Autodesk Fusion 360 part; units mm, degrees
(part 2 of 4)
  spline S79 degree 3 poles (-131.9897, -42.366) (-131.3663, -43.0785) (-131.0085, -44.0182) (-131.0002, -44.9649) (-130.9916, -45.935) (-131.3508, -46.9039) (-131.9897, -47.634) knots -1 -1 -1 -1 -0.506107 -0.506107 -0.506107 0 0 0 0
  spline S80 degree 3 poles (-131.9897, -37.634) (-132.7286, -38.4785) (-133.8364, -38.9881) (-134.9584, -38.9998) (-136.1081, -39.0117) (-137.2531, -38.4994) (-138.0103, -37.634) knots -1 -1 -1 -1 -0.506107 -0.506107 -0.506107 0 0 0 0
  spline S81 degree 3 poles (-138.0103, -37.634) (-138.6337, -36.9215) (-138.9915, -35.9818) (-138.9998, -35.0351) (-139.0084, -34.065) (-138.6492, -33.0961) (-138.0103, -32.366) knots -1 -1 -1 -1 -0.506107 -0.506107 -0.506107 0 0 0 0
  spline S82 degree 3 poles (-138.0103, -32.366) (-137.2714, -31.5215) (-136.1636, -31.0119) (-135.0416, -31.0002) (-133.8919, -30.9883) (-132.7469, -31.5006) (-131.9897, -32.366) knots -1 -1 -1 -1 -0.506107 -0.506107 -0.506107 0 0 0 0
  spline S83 degree 3 poles (-131.9897, -32.366) (-131.3663, -33.0785) (-131.0085, -34.0182) (-131.0002, -34.9649) (-130.9916, -35.935) (-131.3508, -36.9039) (-131.9897, -37.634) knots -1 -1 -1 -1 -0.506107 -0.506107 -0.506107 0 0 0 0
  spline S84 degree 3 poles (-131.9897, -27.634) (-132.7286, -28.4785) (-133.8364, -28.9881) (-134.9584, -28.9998) (-136.1081, -29.0117) (-137.2531, -28.4994) (-138.0103, -27.634) knots -1 -1 -1 -1 -0.506107 -0.506107 -0.506107 0 0 0 0
  spline S85 degree 3 poles (-138.0103, -27.634) (-138.6337, -26.9215) (-138.9915, -25.9818) (-138.9998, -25.0351) (-139.0084, -24.065) (-138.6492, -23.0961) (-138.0103, -22.366) knots -1 -1 -1 -1 -0.506107 -0.506107 -0.506107 0 0 0 0
  spline S86 degree 3 poles (-138.0103, -22.366) (-137.2714, -21.5215) (-136.1636, -21.0119) (-135.0416, -21.0002) (-133.8919, -20.9883) (-132.7469, -21.5006) (-131.9897, -22.366) knots -1 -1 -1 -1 -0.506107 -0.506107 -0.506107 0 0 0 0
  spline S87 degree 3 poles (-131.9897, -22.366) (-131.3663, -23.0785) (-131.0085, -24.0182) (-131.0002, -24.9649) (-130.9916, -25.935) (-131.3508, -26.9039) (-131.9897, -27.634) knots -1 -1 -1 -1 -0.506107 -0.506107 -0.506107 0 0 0 0
  spline S88 degree 3 poles (-131.9897, -17.634) (-132.7286, -18.4785) (-133.8364, -18.9881) (-134.9584, -18.9998) (-136.1081, -19.0117) (-137.2531, -18.4994) (-138.0103, -17.634) knots -1 -1 -1 -1 -0.506107 -0.506107 -0.506107 0 0 0 0
  spline S89 degree 3 poles (-138.0103, -17.634) (-138.6337, -16.9215) (-138.9915, -15.9818) (-138.9998, -15.0351) (-139.0084, -14.065) (-138.6492, -13.0961) (-138.0103, -12.366) knots -1 -1 -1 -1 -0.506107 -0.506107 -0.506107 0 0 0 0
  spline S90 degree 3 poles (-138.0103, -12.366) (-137.2714, -11.5215) (-136.1636, -11.0119) (-135.0416, -11.0002) (-133.8919, -10.9883) (-132.7469, -11.5006) (-131.9897, -12.366) knots -1 -1 -1 -1 -0.506107 -0.506107 -0.506107 0 0 0 0
  spline S91 degree 3 poles (-131.9897, -12.366) (-131.3663, -13.0785) (-131.0085, -14.0182) (-131.0002, -14.9649) (-130.9916, -15.935) (-131.3508, -16.9039) (-131.9897, -17.634) knots -1 -1 -1 -1 -0.506107 -0.506107 -0.506107 0 0 0 0
  spline S92 degree 3 poles (-131.9897, -7.634) (-132.7286, -8.4785) (-133.8364, -8.9881) (-134.9584, -8.9998) (-136.1081, -9.0117) (-137.2531, -8.4994) (-138.0103, -7.634) knots -1 -1 -1 -1 -0.506107 -0.506107 -0.506107 0 0 0 0
  spline S93 degree 3 poles (-138.0103, -7.634) (-138.6337, -6.9215) (-138.9915, -5.9818) (-138.9998, -5.0351) (-139.0084, -4.065) (-138.6492, -3.0961) (-138.0103, -2.366) knots -1 -1 -1 -1 -0.506107 -0.506107 -0.506107 0 0 0 0
  spline S94 degree 3 poles (-138.0103, -2.366) (-137.2714, -1.5215) (-136.1636, -1.0119) (-135.0416, -1.0002) (-133.8919, -0.9883) (-132.7469, -1.5006) (-131.9897, -2.366) knots -1 -1 -1 -1 -0.506107 -0.506107 -0.506107 0 0 0 0
  spline S95 degree 3 poles (-131.9897, -2.366) (-131.3663, -3.0785) (-131.0085, -4.0182) (-131.0002, -4.9649) (-130.9916, -5.935) (-131.3508, -6.9039) (-131.9897, -7.634) knots -1 -1 -1 -1 -0.506107 -0.506107 -0.506107 0 0 0 0
  spline S96 degree 3 poles (-121.9897, -77.634) (-122.7286, -78.4785) (-123.8364, -78.9881) (-124.9584, -78.9998) (-126.1081, -79.0117) (-127.2531, -78.4994) (-128.0103, -77.634) knots -1 -1 -1 -1 -0.506107 -0.506107 -0.506107 0 0 0 0
  spline S97 degree 3 poles (-128.0103, -77.634) (-128.6337, -76.9215) (-128.9915, -75.9818) (-128.9998, -75.0351) (-129.0084, -74.065) (-128.6492, -73.0961) (-128.0103, -72.366) knots -1 -1 -1 -1 -0.506107 -0.506107 -0.506107 0 0 0 0
  spline S98 degree 3 poles (-128.0103, -72.366) (-127.2714, -71.5215) (-126.1636, -71.0119) (-125.0416, -71.0002) (-123.8919, -70.9883) (-122.7469, -71.5006) (-121.9897, -72.366) knots -1 -1 -1 -1 -0.506107 -0.506107 -0.506107 0 0 0 0
  spline S99 degree 3 poles (-121.9897, -72.366) (-121.3663, -73.0785) (-121.0085, -74.0182) (-121.0002, -74.9649) (-120.9916, -75.935) (-121.3508, -76.9039) (-121.9897, -77.634) knots -1 -1 -1 -1 -0.506107 -0.506107 -0.506107 0 0 0 0
  spline S100 degree 3 poles (-121.9897, -67.634) (-122.7286, -68.4785) (-123.8364, -68.9881) (-124.9584, -68.9998) (-126.1081, -69.0117) (-127.2531, -68.4994) (-128.0103, -67.634) knots -1 -1 -1 -1 -0.506107 -0.506107 -0.506107 0 0 0 0
  spline S101 degree 3 poles (-128.0103, -67.634) (-128.6337, -66.9215) (-128.9915, -65.9818) (-128.9998, -65.0351) (-129.0084, -64.065) (-128.6492, -63.0961) (-128.0103, -62.366) knots -1 -1 -1 -1 -0.506107 -0.506107 -0.506107 0 0 0 0
  spline S102 degree 3 poles (-128.0103, -62.366) (-127.2714, -61.5215) (-126.1636, -61.0119) (-125.0416, -61.0002) (-123.8919, -60.9883) (-122.7469, -61.5006) (-121.9897, -62.366) knots -1 -1 -1 -1 -0.506107 -0.506107 -0.506107 0 0 0 0
  spline S103 degree 3 poles (-121.9897, -62.366) (-121.3663, -63.0785) (-121.0085, -64.0182) (-121.0002, -64.9649) (-120.9916, -65.935) (-121.3508, -66.9039) (-121.9897, -67.634) knots -1 -1 -1 -1 -0.506107 -0.506107 -0.506107 0 0 0 0
  spline S104 degree 3 poles (-121.9897, -57.634) (-122.7286, -58.4785) (-123.8364, -58.9881) (-124.9584, -58.9998) (-126.1081, -59.0117) (-127.2531, -58.4994) (-128.0103, -57.634) knots -1 -1 -1 -1 -0.506107 -0.506107 -0.506107 0 0 0 0
  spline S105 degree 3 poles (-128.0103, -57.634) (-128.6337, -56.9215) (-128.9915, -55.9818) (-128.9998, -55.0351) (-129.0084, -54.065) (-128.6492, -53.0961) (-128.0103, -52.366) knots -1 -1 -1 -1 -0.506107 -0.506107 -0.506107 0 0 0 0
  spline S106 degree 3 poles (-128.0103, -52.366) (-127.2714, -51.5215) (-126.1636, -51.0119) (-125.0416, -51.0002) (-123.8919, -50.9883) (-122.7469, -51.5006) (-121.9897, -52.366) knots -1 -1 -1 -1 -0.506107 -0.506107 -0.506107 0 0 0 0
  spline S107 degree 3 poles (-121.9897, -52.366) (-121.3663, -53.0785) (-121.0085, -54.0182) (-121.0002, -54.9649) (-120.9916, -55.935) (-121.3508, -56.9039) (-121.9897, -57.634) knots -1 -1 -1 -1 -0.506107 -0.506107 -0.506107 0 0 0 0
  spline S108 degree 3 poles (-121.9897, -47.634) (-122.7286, -48.4785) (-123.8364, -48.9881) (-124.9584, -48.9998) (-126.1081, -49.0117) (-127.2531, -48.4994) (-128.0103, -47.634) knots -1 -1 -1 -1 -0.506107 -0.506107 -0.506107 0 0 0 0
  spline S109 degree 3 poles (-128.0103, -47.634) (-128.6337, -46.9215) (-128.9915, -45.9818) (-128.9998, -45.0351) (-129.0084, -44.065) (-128.6492, -43.0961) (-128.0103, -42.366) knots -1 -1 -1 -1 -0.506107 -0.506107 -0.506107 0 0 0 0
  spline S110 degree 3 poles (-128.0103, -42.366) (-127.2714, -41.5215) (-126.1636, -41.0119) (-125.0416, -41.0002) (-123.8919, -40.9883) (-122.7469, -41.5006) (-121.9897, -42.366) knots -1 -1 -1 -1 -0.506107 -0.506107 -0.506107 0 0 0 0
  spline S111 degree 3 poles (-121.9897, -42.366) (-121.3663, -43.0785) (-121.0085, -44.0182) (-121.0002, -44.9649) (-120.9916, -45.935) (-121.3508, -46.9039) (-121.9897, -47.634) knots -1 -1 -1 -1 -0.506107 -0.506107 -0.506107 0 0 0 0
  spline S112 degree 3 poles (-121.9897, -37.634) (-122.7286, -38.4785) (-123.8364, -38.9881) (-124.9584, -38.9998) (-126.1081, -39.0117) (-127.2531, -38.4994) (-128.0103, -37.634) knots -1 -1 -1 -1 -0.506107 -0.506107 -0.506107 0 0 0 0
  spline S113 degree 3 poles (-128.0103, -37.634) (-128.6337, -36.9215) (-128.9915, -35.9818) (-128.9998, -35.0351) (-129.0084, -34.065) (-128.6492, -33.0961) (-128.0103, -32.366) knots -1 -1 -1 -1 -0.506107 -0.506107 -0.506107 0 0 0 0
  spline S114 degree 3 poles (-128.0103, -32.366) (-127.2714, -31.5215) (-126.1636, -31.0119) (-125.0416, -31.0002) (-123.8919, -30.9883) (-122.7469, -31.5006) (-121.9897, -32.366) knots -1 -1 -1 -1 -0.506107 -0.506107 -0.506107 0 0 0 0
  spline S115 degree 3 poles (-121.9897, -32.366) (-121.3663, -33.0785) (-121.0085, -34.0182) (-121.0002, -34.9649) (-120.9916, -35.935) (-121.3508, -36.9039) (-121.9897, -37.634) knots -1 -1 -1 -1 -0.506107 -0.506107 -0.506107 0 0 0 0
  spline S116 degree 3 poles (-121.9897, -27.634) (-122.7286, -28.4785) (-123.8364, -28.9881) (-124.9584, -28.9998) (-126.1081, -29.0117) (-127.2531, -28.4994) (-128.0103, -27.634) knots -1 -1 -1 -1 -0.506107 -0.506107 -0.506107 0 0 0 0
  spline S117 degree 3 poles (-128.0103, -27.634) (-128.6337, -26.9215) (-128.9915, -25.9818) (-128.9998, -25.0351) (-129.0084, -24.065) (-128.6492, -23.0961) (-128.0103, -22.366) knots -1 -1 -1 -1 -0.506107 -0.506107 -0.506107 0 0 0 0
  spline S118 degree 3 poles (-128.0103, -22.366) (-127.2714, -21.5215) (-126.1636, -21.0119) (-125.0416, -21.0002) (-123.8919, -20.9883) (-122.7469, -21.5006) (-121.9897, -22.366) knots -1 -1 -1 -1 -0.506107 -0.506107 -0.506107 0 0 0 0
  spline S119 degree 3 poles (-121.9897, -22.366) (-121.3663, -23.0785) (-121.0085, -24.0182) (-121.0002, -24.9649) (-120.9916, -25.935) (-121.3508, -26.9039) (-121.9897, -27.634) knots -1 -1 -1 -1 -0.506107 -0.506107 -0.506107 0 0 0 0
  spline S120 degree 3 poles (-121.9897, -17.634) (-122.7286, -18.4785) (-123.8364, -18.9881) (-124.9584, -18.9998) (-126.1081, -19.0117) (-127.2531, -18.4994) (-128.0103, -17.634) knots -1 -1 -1 -1 -0.506107 -0.506107 -0.506107 0 0 0 0
  spline S121 degree 3 poles (-128.0103, -17.634) (-128.6337, -16.9215) (-128.9915, -15.9818) (-128.9998, -15.0351) (-129.0084, -14.065) (-128.6492, -13.0961) (-128.0103, -12.366) knots -1 -1 -1 -1 -0.506107 -0.506107 -0.506107 0 0 0 0
  spline S122 degree 3 poles (-128.0103, -12.366) (-127.2714, -11.5215) (-126.1636, -11.0119) (-125.0416, -11.0002) (-123.8919, -10.9883) (-122.7469, -11.5006) (-121.9897, -12.366) knots -1 -1 -1 -1 -0.506107 -0.506107 -0.506107 0 0 0 0
  spline S123 degree 3 poles (-121.9897, -12.366) (-121.3663, -13.0785) (-121.0085, -14.0182) (-121.0002, -14.9649) (-120.9916, -15.935) (-121.3508, -16.9039) (-121.9897, -17.634) knots -1 -1 -1 -1 -0.506107 -0.506107 -0.506107 0 0 0 0
  spline S124 degree 3 poles (-121.9897, -7.634) (-122.7286, -8.4785) (-123.8364, -8.9881) (-124.9584, -8.9998) (-126.1081, -9.0117) (-127.2531, -8.4994) (-128.0103, -7.634) knots -1 -1 -1 -1 -0.506107 -0.506107 -0.506107 0 0 0 0
  spline S125 degree 3 poles (-128.0103, -7.634) (-128.6337, -6.9215) (-128.9915, -5.9818) (-128.9998, -5.0351) (-129.0084, -4.065) (-128.6492, -3.0961) (-128.0103, -2.366) knots -1 -1 -1 -1 -0.506107 -0.506107 -0.506107 0 0 0 0
  spline S126 degree 3 poles (-128.0103, -2.366) (-127.2714, -1.5215) (-126.1636, -1.0119) (-125.0416, -1.0002) (-123.8919, -0.9883) (-122.7469, -1.5006) (-121.9897, -2.366) knots -1 -1 -1 -1 -0.506107 -0.506107 -0.506107 0 0 0 0
  spline S127 degree 3 poles (-121.9897, -2.366) (-121.3663, -3.0785) (-121.0085, -4.0182) (-121.0002, -4.9649) (-120.9916, -5.935) (-121.3508, -6.9039) (-121.9897, -7.634) knots -1 -1 -1 -1 -0.506107 -0.506107 -0.506107 0 0 0 0
  spline S128 degree 3 poles (-111.9897, -77.634) (-112.7286, -78.4785) (-113.8364, -78.9881) (-114.9584, -78.9998) (-116.1081, -79.0117) (-117.2531, -78.4994) (-118.0103, -77.634) knots -1 -1 -1 -1 -0.506107 -0.506107 -0.506107 0 0 0 0
  spline S129 degree 3 poles (-118.0103, -77.634) (-118.6337, -76.9215) (-118.9915, -75.9818) (-118.9998, -75.0351) (-119.0084, -74.065) (-118.6492, -73.0961) (-118.0103, -72.366) knots -1 -1 -1 -1 -0.506107 -0.506107 -0.506107 0 0 0 0
  spline S130 degree 3 poles (-118.0103, -72.366) (-117.2714, -71.5215) (-116.1636, -71.0119) (-115.0416, -71.0002) (-113.8919, -70.9883) (-112.7469, -71.5006) (-111.9897, -72.366) knots -1 -1 -1 -1 -0.506107 -0.506107 -0.506107 0 0 0 0
  spline S131 degree 3 poles (-111.9897, -72.366) (-111.3663, -73.0785) (-111.0085, -74.0182) (-111.0002, -74.9649) (-110.9916, -75.935) (-111.3508, -76.9039) (-111.9897, -77.634) knots -1 -1 -1 -1 -0.506107 -0.506107 -0.506107 0 0 0 0
  spline S132 degree 3 poles (-111.9897, -67.634) (-112.7286, -68.4785) (-113.8364, -68.9881) (-114.9584, -68.9998) (-116.1081, -69.0117) (-117.2531, -68.4994) (-118.0103, -67.634) knots -1 -1 -1 -1 -0.506107 -0.506107 -0.506107 0 0 0 0
  spline S133 degree 3 poles (-118.0103, -67.634) (-118.6337, -66.9215) (-118.9915, -65.9818) (-118.9998, -65.0351) (-119.0084, -64.065) (-118.6492, -63.0961) (-118.0103, -62.366) knots -1 -1 -1 -1 -0.506107 -0.506107 -0.506107 0 0 0 0
  spline S134 degree 3 poles (-118.0103, -62.366) (-117.2714, -61.5215) (-116.1636, -61.0119) (-115.0416, -61.0002) (-113.8919, -60.9883) (-112.7469, -61.5006) (-111.9897, -62.366) knots -1 -1 -1 -1 -0.506107 -0.506107 -0.506107 0 0 0 0
  spline S135 degree 3 poles (-111.9897, -62.366) (-111.3663, -63.0785) (-111.0085, -64.0182) (-111.0002, -64.9649) (-110.9916, -65.935) (-111.3508, -66.9039) (-111.9897, -67.634) knots -1 -1 -1 -1 -0.506107 -0.506107 -0.506107 0 0 0 0
  spline S136 degree 3 poles (-111.9897, -57.634) (-112.7286, -58.4785) (-113.8364, -58.9881) (-114.9584, -58.9998) (-116.1081, -59.0117) (-117.2531, -58.4994) (-118.0103, -57.634) knots -1 -1 -1 -1 -0.506107 -0.506107 -0.506107 0 0 0 0
  spline S137 degree 3 poles (-118.0103, -57.634) (-118.6337, -56.9215) (-118.9915, -55.9818) (-118.9998, -55.0351) (-119.0084, -54.065) (-118.6492, -53.0961) (-118.0103, -52.366) knots -1 -1 -1 -1 -0.506107 -0.506107 -0.506107 0 0 0 0
  spline S138 degree 3 poles (-118.0103, -52.366) (-117.2714, -51.5215) (-116.1636, -51.0119) (-115.0416, -51.0002) (-113.8919, -50.9883) (-112.7469, -51.5006) (-111.9897, -52.366) knots -1 -1 -1 -1 -0.506107 -0.506107 -0.506107 0 0 0 0
  spline S139 degree 3 poles (-111.9897, -52.366) (-111.3663, -53.0785) (-111.0085, -54.0182) (-111.0002, -54.9649) (-110.9916, -55.935) (-111.3508, -56.9039) (-111.9897, -57.634) knots -1 -1 -1 -1 -0.506107 -0.506107 -0.506107 0 0 0 0
  spline S140 degree 3 poles (-111.9897, -47.634) (-112.7286, -48.4785) (-113.8364, -48.9881) (-114.9584, -48.9998) (-116.1081, -49.0117) (-117.2531, -48.4994) (-118.0103, -47.634) knots -1 -1 -1 -1 -0.506107 -0.506107 -0.506107 0 0 0 0
  spline S141 degree 3 poles (-118.0103, -47.634) (-118.6337, -46.9215) (-118.9915, -45.9818) (-118.9998, -45.0351) (-119.0084, -44.065) (-118.6492, -43.0961) (-118.0103, -42.366) knots -1 -1 -1 -1 -0.506107 -0.506107 -0.506107 0 0 0 0
  spline S142 degree 3 poles (-118.0103, -42.366) (-117.2714, -41.5215) (-116.1636, -41.0119) (-115.0416, -41.0002) (-113.8919, -40.9883) (-112.7469, -41.5006) (-111.9897, -42.366) knots -1 -1 -1 -1 -0.506107 -0.506107 -0.506107 0 0 0 0
  spline S143 degree 3 poles (-111.9897, -42.366) (-111.3663, -43.0785) (-111.0085, -44.0182) (-111.0002, -44.9649) (-110.9916, -45.935) (-111.3508, -46.9039) (-111.9897, -47.634) knots -1 -1 -1 -1 -0.506107 -0.506107 -0.506107 0 0 0 0
  spline S144 degree 3 poles (-111.9897, -37.634) (-112.7286, -38.4785) (-113.8364, -38.9881) (-114.9584, -38.9998) (-116.1081, -39.0117) (-117.2531, -38.4994) (-118.0103, -37.634) knots -1 -1 -1 -1 -0.506107 -0.506107 -0.506107 0 0 0 0
  spline S145 degree 3 poles (-118.0103, -37.634) (-118.6337, -36.9215) (-118.9915, -35.9818) (-118.9998, -35.0351) (-119.0084, -34.065) (-118.6492, -33.0961) (-118.0103, -32.366) knots -1 -1 -1 -1 -0.506107 -0.506107 -0.506107 0 0 0 0
  spline S146 degree 3 poles (-118.0103, -32.366) (-117.2714, -31.5215) (-116.1636, -31.0119) (-115.0416, -31.0002) (-113.8919, -30.9883) (-112.7469, -31.5006) (-111.9897, -32.366) knots -1 -1 -1 -1 -0.506107 -0.506107 -0.506107 0 0 0 0
  spline S147 degree 3 poles (-111.9897, -32.366) (-111.3663, -33.0785) (-111.0085, -34.0182) (-111.0002, -34.9649) (-110.9916, -35.935) (-111.3508, -36.9039) (-111.9897, -37.634) knots -1 -1 -1 -1 -0.506107 -0.506107 -0.506107 0 0 0 0
  spline S148 degree 3 poles (-111.9897, -27.634) (-112.7286, -28.4785) (-113.8364, -28.9881) (-114.9584, -28.9998) (-116.1081, -29.0117) (-117.2531, -28.4994) (-118.0103, -27.634) knots -1 -1 -1 -1 -0.506107 -0.506107 -0.506107 0 0 0 0
  spline S149 degree 3 poles (-118.0103, -27.634) (-118.6337, -26.9215) (-118.9915, -25.9818) (-118.9998, -25.0351) (-119.0084, -24.065) (-118.6492, -23.0961) (-118.0103, -22.366) knots -1 -1 -1 -1 -0.506107 -0.506107 -0.506107 0 0 0 0
  spline S150 degree 3 poles (-118.0103, -22.366) (-117.2714, -21.5215) (-116.1636, -21.0119) (-115.0416, -21.0002) (-113.8919, -20.9883) (-112.7469, -21.5006) (-111.9897, -22.366) knots -1 -1 -1 -1 -0.506107 -0.506107 -0.506107 0 0 0 0
  spline S151 degree 3 poles (-111.9897, -22.366) (-111.3663, -23.0785) (-111.0085, -24.0182) (-111.0002, -24.9649) (-110.9916, -25.935) (-111.3508, -26.9039) (-111.9897, -27.634) knots -1 -1 -1 -1 -0.506107 -0.506107 -0.506107 0 0 0 0
  spline S152 degree 3 poles (-111.9897, -17.634) (-112.7286, -18.4785) (-113.8364, -18.9881) (-114.9584, -18.9998) (-116.1081, -19.0117) (-117.2531, -18.4994) (-118.0103, -17.634) knots -1 -1 -1 -1 -0.506107 -0.506107 -0.506107 0 0 0 0
  spline S153 degree 3 poles (-118.0103, -17.634) (-118.6337, -16.9215) (-118.9915, -15.9818) (-118.9998, -15.0351) (-119.0084, -14.065) (-118.6492, -13.0961) (-118.0103, -12.366) knots -1 -1 -1 -1 -0.506107 -0.506107 -0.506107 0 0 0 0
  spline S154 degree 3 poles (-118.0103, -12.366) (-117.2714, -11.5215) (-116.1636, -11.0119) (-115.0416, -11.0002) (-113.8919, -10.9883) (-112.7469, -11.5006) (-111.9897, -12.366) knots -1 -1 -1 -1 -0.506107 -0.506107 -0.506107 0 0 0 0
  spline S155 degree 3 poles (-111.9897, -12.366) (-111.3663, -13.0785) (-111.0085, -14.0182) (-111.0002, -14.9649) (-110.9916, -15.935) (-111.3508, -16.9039) (-111.9897, -17.634) knots -1 -1 -1 -1 -0.506107 -0.506107 -0.506107 0 0 0 0
  spline S156 degree 3 poles (-111.9897, -7.634) (-112.7286, -8.4785) (-113.8364, -8.9881) (-114.9584, -8.9998) (-116.1081, -9.0117) (-117.2531, -8.4994) (-118.0103, -7.634) knots -1 -1 -1 -1 -0.506107 -0.506107 -0.506107 0 0 0 0
  spline S157 degree 3 poles (-118.0103, -7.634) (-118.6337, -6.9215) (-118.9915, -5.9818) (-118.9998, -5.0351) (-119.0084, -4.065) (-118.6492, -3.0961) (-118.0103, -2.366) knots -1 -1 -1 -1 -0.506107 -0.506107 -0.506107 0 0 0 0
  spline S158 degree 3 poles (-118.0103, -2.366) (-117.2714, -1.5215) (-116.1636, -1.0119) (-115.0416, -1.0002) (-113.8919, -0.9883) (-112.7469, -1.5006) (-111.9897, -2.366) knots -1 -1 -1 -1 -0.506107 -0.506107 -0.506107 0 0 0 0
  spline S159 degree 3 poles (-111.9897, -2.366) (-111.3663, -3.0785) (-111.0085, -4.0182) (-111.0002, -4.9649) (-110.9916, -5.935) (-111.3508, -6.9039) (-111.9897, -7.634) knots -1 -1 -1 -1 -0.506107 -0.506107 -0.506107 0 0 0 0
  spline S160 degree 3 poles (-101.9897, -77.634) (-102.7286, -78.4785) (-103.8364, -78.9881) (-104.9584, -78.9998) (-106.1081, -79.0117) (-107.2531, -78.4994) (-108.0103, -77.634) knots -1 -1 -1 -1 -0.506107 -0.506107 -0.506107 0 0 0 0
  spline S161 degree 3 poles (-108.0103, -77.634) (-108.6337, -76.9215) (-108.9915, -75.9818) (-108.9998, -75.0351) (-109.0084, -74.065) (-108.6492, -73.0961) (-108.0103, -72.366) knots -1 -1 -1 -1 -0.506107 -0.506107 -0.506107 0 0 0 0
  spline S162 degree 3 poles (-108.0103, -72.366) (-107.2714, -71.5215) (-106.1636, -71.0119) (-105.0416, -71.0002) (-103.8919, -70.9883) (-102.7469, -71.5006) (-101.9897, -72.366) knots -1 -1 -1 -1 -0.506107 -0.506107 -0.506107 0 0 0 0
  spline S163 degree 3 poles (-101.9897, -72.366) (-101.3663, -73.0785) (-101.0085, -74.0182) (-101.0002, -74.9649) (-100.9916, -75.935) (-101.3508, -76.9039) (-101.9897, -77.634) knots -1 -1 -1 -1 -0.506107 -0.506107 -0.506107 0 0 0 0
  spline S164 degree 3 poles (-101.9897, -67.634) (-102.7286, -68.4785) (-103.8364, -68.9881) (-104.9584, -68.9998) (-106.1081, -69.0117) (-107.2531, -68.4994) (-108.0103, -67.634) knots -1 -1 -1 -1 -0.506107 -0.506107 -0.506107 0 0 0 0
  spline S165 degree 3 poles (-108.0103, -67.634) (-108.6337, -66.9215) (-108.9915, -65.9818) (-108.9998, -65.0351) (-109.0084, -64.065) (-108.6492, -63.0961) (-108.0103, -62.366) knots -1 -1 -1 -1 -0.506107 -0.506107 -0.506107 0 0 0 0
  spline S166 degree 3 poles (-108.0103, -62.366) (-107.2714, -61.5215) (-106.1636, -61.0119) (-105.0416, -61.0002) (-103.8919, -60.9883) (-102.7469, -61.5006) (-101.9897, -62.366) knots -1 -1 -1 -1 -0.506107 -0.506107 -0.506107 0 0 0 0
  spline S167 degree 3 poles (-101.9897, -62.366) (-101.3663, -63.0785) (-101.0085, -64.0182) (-101.0002, -64.9649) (-100.9916, -65.935) (-101.3508, -66.9039) (-101.9897, -67.634) knots -1 -1 -1 -1 -0.506107 -0.506107 -0.506107 0 0 0 0
  spline S168 degree 3 poles (-101.9897, -57.634) (-102.7286, -58.4785) (-103.8364, -58.9881) (-104.9584, -58.9998) (-106.1081, -59.0117) (-107.2531, -58.4994) (-108.0103, -57.634) knots -1 -1 -1 -1 -0.506107 -0.506107 -0.506107 0 0 0 0
  spline S169 degree 3 poles (-108.0103, -57.634) (-108.6337, -56.9215) (-108.9915, -55.9818) (-108.9998, -55.0351) (-109.0084, -54.065) (-108.6492, -53.0961) (-108.0103, -52.366) knots -1 -1 -1 -1 -0.506107 -0.506107 -0.506107 0 0 0 0
  spline S170 degree 3 poles (-108.0103, -52.366) (-107.2714, -51.5215) (-106.1636, -51.0119) (-105.0416, -51.0002) (-103.8919, -50.9883) (-102.7469, -51.5006) (-101.9897, -52.366) knots -1 -1 -1 -1 -0.506107 -0.506107 -0.506107 0 0 0 0
  spline S171 degree 3 poles (-101.9897, -52.366) (-101.3663, -53.0785) (-101.0085, -54.0182) (-101.0002, -54.9649) (-100.9916, -55.935) (-101.3508, -56.9039) (-101.9897, -57.634) knots -1 -1 -1 -1 -0.506107 -0.506107 -0.506107 0 0 0 0
  spline S172 degree 3 poles (-101.9897, -47.634) (-102.7286, -48.4785) (-103.8364, -48.9881) (-104.9584, -48.9998) (-106.1081, -49.0117) (-107.2531, -48.4994) (-108.0103, -47.634) knots -1 -1 -1 -1 -0.506107 -0.506107 -0.506107 0 0 0 0
  spline S173 degree 3 poles (-108.0103, -47.634) (-108.6337, -46.9215) (-108.9915, -45.9818) (-108.9998, -45.0351) (-109.0084, -44.065) (-108.6492, -43.0961) (-108.0103, -42.366) knots -1 -1 -1 -1 -0.506107 -0.506107 -0.506107 0 0 0 0
  spline S174 degree 3 poles (-108.0103, -42.366) (-107.2714, -41.5215) (-106.1636, -41.0119) (-105.0416, -41.0002) (-103.8919, -40.9883) (-102.7469, -41.5006) (-101.9897, -42.366) knots -1 -1 -1 -1 -0.506107 -0.506107 -0.506107 0 0 0 0
  spline S175 degree 3 poles (-101.9897, -42.366) (-101.3663, -43.0785) (-101.0085, -44.0182) (-101.0002, -44.9649) (-100.9916, -45.935) (-101.3508, -46.9039) (-101.9897, -47.634) knots -1 -1 -1 -1 -0.506107 -0.506107 -0.506107 0 0 0 0
  spline S176 degree 3 poles (-101.9897, -37.634) (-102.7286, -38.4785) (-103.8364, -38.9881) (-104.9584, -38.9998) (-106.1081, -39.0117) (-107.2531, -38.4994) (-108.0103, -37.634) knots -1 -1 -1 -1 -0.506107 -0.506107 -0.506107 0 0 0 0
  spline S177 degree 3 poles (-108.0103, -37.634) (-108.6337, -36.9215) (-108.9915, -35.9818) (-108.9998, -35.0351) (-109.0084, -34.065) (-108.6492, -33.0961) (-108.0103, -32.366) knots -1 -1 -1 -1 -0.506107 -0.506107 -0.506107 0 0 0 0
  spline S178 degree 3 poles (-108.0103, -32.366) (-107.2714, -31.5215) (-106.1636, -31.0119) (-105.0416, -31.0002) (-103.8919, -30.9883) (-102.7469, -31.5006) (-101.9897, -32.366) knots -1 -1 -1 -1 -0.506107 -0.506107 -0.506107 0 0 0 0
  spline S179 degree 3 poles (-101.9897, -32.366) (-101.3663, -33.0785) (-101.0085, -34.0182) (-101.0002, -34.9649) (-100.9916, -35.935) (-101.3508, -36.9039) (-101.9897, -37.634) knots -1 -1 -1 -1 -0.506107 -0.506107 -0.506107 0 0 0 0
  spline S180 degree 3 poles (-101.9897, -27.634) (-102.7286, -28.4785) (-103.8364, -28.9881) (-104.9584, -28.9998) (-106.1081, -29.0117) (-107.2531, -28.4994) (-108.0103, -27.634) knots -1 -1 -1 -1 -0.506107 -0.506107 -0.506107 0 0 0 0
  spline S181 degree 3 poles (-108.0103, -27.634) (-108.6337, -26.9215) (-108.9915, -25.9818) (-108.9998, -25.0351) (-109.0084, -24.065) (-108.6492, -23.0961) (-108.0103, -22.366) knots -1 -1 -1 -1 -0.506107 -0.506107 -0.506107 0 0 0 0
  spline S182 degree 3 poles (-108.0103, -22.366) (-107.2714, -21.5215) (-106.1636, -21.0119) (-105.0416, -21.0002) (-103.8919, -20.9883) (-102.7469, -21.5006) (-101.9897, -22.366) knots -1 -1 -1 -1 -0.506107 -0.506107 -0.506107 0 0 0 0
  spline S183 degree 3 poles (-101.9897, -22.366) (-101.3663, -23.0785) (-101.0085, -24.0182) (-101.0002, -24.9649) (-100.9916, -25.935) (-101.3508, -26.9039) (-101.9897, -27.634) knots -1 -1 -1 -1 -0.506107 -0.506107 -0.506107 0 0 0 0
  spline S184 degree 3 poles (-101.9897, -17.634) (-102.7286, -18.4785) (-103.8364, -18.9881) (-104.9584, -18.9998) (-106.1081, -19.0117) (-107.2531, -18.4994) (-108.0103, -17.634) knots -1 -1 -1 -1 -0.506107 -0.506107 -0.506107 0 0 0 0
  spline S185 degree 3 poles (-108.0103, -17.634) (-108.6337, -16.9215) (-108.9915, -15.9818) (-108.9998, -15.0351) (-109.0084, -14.065) (-108.6492, -13.0961) (-108.0103, -12.366) knots -1 -1 -1 -1 -0.506107 -0.506107 -0.506107 0 0 0 0
  spline S186 degree 3 poles (-108.0103, -12.366) (-107.2714, -11.5215) (-106.1636, -11.0119) (-105.0416, -11.0002) (-103.8919, -10.9883) (-102.7469, -11.5006) (-101.9897, -12.366) knots -1 -1 -1 -1 -0.506107 -0.506107 -0.506107 0 0 0 0
  spline S187 degree 3 poles (-101.9897, -12.366) (-101.3663, -13.0785) (-101.0085, -14.0182) (-101.0002, -14.9649) (-100.9916, -15.935) (-101.3508, -16.9039) (-101.9897, -17.634) knots -1 -1 -1 -1 -0.506107 -0.506107 -0.506107 0 0 0 0
  spline S188 degree 3 poles (-101.9897, -7.634) (-102.7286, -8.4785) (-103.8364, -8.9881) (-104.9584, -8.9998) (-106.1081, -9.0117) (-107.2531, -8.4994) (-108.0103, -7.634) knots -1 -1 -1 -1 -0.506107 -0.506107 -0.506107 0 0 0 0
  spline S189 degree 3 poles (-108.0103, -7.634) (-108.6337, -6.9215) (-108.9915, -5.9818) (-108.9998, -5.0351) (-109.0084, -4.065) (-108.6492, -3.0961) (-108.0103, -2.366) knots -1 -1 -1 -1 -0.506107 -0.506107 -0.506107 0 0 0 0
  spline S190 degree 3 poles (-108.0103, -2.366) (-107.2714, -1.5215) (-106.1636, -1.0119) (-105.0416, -1.0002) (-103.8919, -0.9883) (-102.7469, -1.5006) (-101.9897, -2.366) knots -1 -1 -1 -1 -0.506107 -0.506107 -0.506107 0 0 0 0
  spline S191 degree 3 poles (-101.9897, -2.366) (-101.3663, -3.0785) (-101.0085, -4.0182) (-101.0002, -4.9649) (-100.9916, -5.935) (-101.3508, -6.9039) (-101.9897, -7.634) knots -1 -1 -1 -1 -0.506107 -0.506107 -0.506107 0 0 0 0
  spline S192 degree 3 poles (-91.9897, -77.634) (-92.7286, -78.4785) (-93.8364, -78.9881) (-94.9584, -78.9998) (-96.1081, -79.0117) (-97.2531, -78.4994) (-98.0103, -77.634) knots -1 -1 -1 -1 -0.506107 -0.506107 -0.506107 0 0 0 0
  spline S193 degree 3 poles (-98.0103, -77.634) (-98.6337, -76.9215) (-98.9915, -75.9818) (-98.9998, -75.0351) (-99.0084, -74.065) (-98.6492, -73.0961) (-98.0103, -72.366) knots -1 -1 -1 -1 -0.506107 -0.506107 -0.506107 0 0 0 0
  spline S194 degree 3 poles (-98.0103, -72.366) (-97.2714, -71.5215) (-96.1636, -71.0119) (-95.0416, -71.0002) (-93.8919, -70.9883) (-92.7469, -71.5006) (-91.9897, -72.366) knots -1 -1 -1 -1 -0.506107 -0.506107 -0.506107 0 0 0 0
  spline S195 degree 3 poles (-91.9897, -72.366) (-91.3663, -73.0785) (-91.0085, -74.0182) (-91.0002, -74.9649) (-90.9916, -75.935) (-91.3508, -76.9039) (-91.9897, -77.634) knots -1 -1 -1 -1 -0.506107 -0.506107 -0.506107 0 0 0 0
  spline S196 degree 3 poles (-91.9897, -67.634) (-92.7286, -68.4785) (-93.8364, -68.9881) (-94.9584, -68.9998) (-96.1081, -69.0117) (-97.2531, -68.4994) (-98.0103, -67.634) knots -1 -1 -1 -1 -0.506107 -0.506107 -0.506107 0 0 0 0
  spline S197 degree 3 poles (-98.0103, -67.634) (-98.6337, -66.9215) (-98.9915, -65.9818) (-98.9998, -65.0351) (-99.0084, -64.065) (-98.6492, -63.0961) (-98.0103, -62.366) knots -1 -1 -1 -1 -0.506107 -0.506107 -0.506107 0 0 0 0
  spline S198 degree 3 poles (-98.0103, -62.366) (-97.2714, -61.5215) (-96.1636, -61.0119) (-95.0416, -61.0002) (-93.8919, -60.9883) (-92.7469, -61.5006) (-91.9897, -62.366) knots -1 -1 -1 -1 -0.506107 -0.506107 -0.506107 0 0 0 0
  spline S199 degree 3 poles (-91.9897, -62.366) (-91.3663, -63.0785) (-91.0085, -64.0182) (-91.0002, -64.9649) (-90.9916, -65.935) (-91.3508, -66.9039) (-91.9897, -67.634) knots -1 -1 -1 -1 -0.506107 -0.506107 -0.506107 0 0 0 0
  spline S200 degree 3 poles (-91.9897, -57.634) (-92.7286, -58.4785) (-93.8364, -58.9881) (-94.9584, -58.9998) (-96.1081, -59.0117) (-97.2531, -58.4994) (-98.0103, -57.634) knots -1 -1 -1 -1 -0.506107 -0.506107 -0.506107 0 0 0 0
  spline S201 degree 3 poles (-98.0103, -57.634) (-98.6337, -56.9215) (-98.9915, -55.9818) (-98.9998, -55.0351) (-99.0084, -54.065) (-98.6492, -53.0961) (-98.0103, -52.366) knots -1 -1 -1 -1 -0.506107 -0.506107 -0.506107 0 0 0 0
  spline S202 degree 3 poles (-98.0103, -52.366) (-97.2714, -51.5215) (-96.1636, -51.0119) (-95.0416, -51.0002) (-93.8919, -50.9883) (-92.7469, -51.5006) (-91.9897, -52.366) knots -1 -1 -1 -1 -0.506107 -0.506107 -0.506107 0 0 0 0
  spline S203 degree 3 poles (-91.9897, -52.366) (-91.3663, -53.0785) (-91.0085, -54.0182) (-91.0002, -54.9649) (-90.9916, -55.935) (-91.3508, -56.9039) (-91.9897, -57.634) knots -1 -1 -1 -1 -0.506107 -0.506107 -0.506107 0 0 0 0
  spline S204 degree 3 poles (-91.9897, -47.634) (-92.7286, -48.4785) (-93.8364, -48.9881) (-94.9584, -48.9998) (-96.1081, -49.0117) (-97.2531, -48.4994) (-98.0103, -47.634) knots -1 -1 -1 -1 -0.506107 -0.506107 -0.506107 0 0 0 0
  spline S205 degree 3 poles (-98.0103, -47.634) (-98.6337, -46.9215) (-98.9915, -45.9818) (-98.9998, -45.0351) (-99.0084, -44.065) (-98.6492, -43.0961) (-98.0103, -42.366) knots -1 -1 -1 -1 -0.506107 -0.506107 -0.506107 0 0 0 0
  spline S206 degree 3 poles (-98.0103, -42.366) (-97.2714, -41.5215) (-96.1636, -41.0119) (-95.0416, -41.0002) (-93.8919, -40.9883) (-92.7469, -41.5006) (-91.9897, -42.366) knots -1 -1 -1 -1 -0.506107 -0.506107 -0.506107 0 0 0 0
  spline S207 degree 3 poles (-91.9897, -42.366) (-91.3663, -43.0785) (-91.0085, -44.0182) (-91.0002, -44.9649) (-90.9916, -45.935) (-91.3508, -46.9039) (-91.9897, -47.634) knots -1 -1 -1 -1 -0.506107 -0.506107 -0.506107 0 0 0 0
  spline S208 degree 3 poles (-91.9897, -37.634) (-92.7286, -38.4785) (-93.8364, -38.9881) (-94.9584, -38.9998) (-96.1081, -39.0117) (-97.2531, -38.4994) (-98.0103, -37.634) knots -1 -1 -1 -1 -0.506107 -0.506107 -0.506107 0 0 0 0
  spline S209 degree 3 poles (-98.0103, -37.634) (-98.6337, -36.9215) (-98.9915, -35.9818) (-98.9998, -35.0351) (-99.0084, -34.065) (-98.6492, -33.0961) (-98.0103, -32.366) knots -1 -1 -1 -1 -0.506107 -0.506107 -0.506107 0 0 0 0
  spline S210 degree 3 poles (-98.0103, -32.366) (-97.2714, -31.5215) (-96.1636, -31.0119) (-95.0416, -31.0002) (-93.8919, -30.9883) (-92.7469, -31.5006) (-91.9897, -32.366) knots -1 -1 -1 -1 -0.506107 -0.506107 -0.506107 0 0 0 0
  spline S211 degree 3 poles (-91.9897, -32.366) (-91.3663, -33.0785) (-91.0085, -34.0182) (-91.0002, -34.9649) (-90.9916, -35.935) (-91.3508, -36.9039) (-91.9897, -37.634) knots -1 -1 -1 -1 -0.506107 -0.506107 -0.506107 0 0 0 0
  spline S212 degree 3 poles (-91.9897, -27.634) (-92.7286, -28.4785) (-93.8364, -28.9881) (-94.9584, -28.9998) (-96.1081, -29.0117) (-97.2531, -28.4994) (-98.0103, -27.634) knots -1 -1 -1 -1 -0.506107 -0.506107 -0.506107 0 0 0 0
  spline S213 degree 3 poles (-98.0103, -27.634) (-98.6337, -26.9215) (-98.9915, -25.9818) (-98.9998, -25.0351) (-99.0084, -24.065) (-98.6492, -23.0961) (-98.0103, -22.366) knots -1 -1 -1 -1 -0.506107 -0.506107 -0.506107 0 0 0 0
  spline S214 degree 3 poles (-98.0103, -22.366) (-97.2714, -21.5215) (-96.1636, -21.0119) (-95.0416, -21.0002) (-93.8919, -20.9883) (-92.7469, -21.5006) (-91.9897, -22.366) knots -1 -1 -1 -1 -0.506107 -0.506107 -0.506107 0 0 0 0
  spline S215 degree 3 poles (-91.9897, -22.366) (-91.3663, -23.0785) (-91.0085, -24.0182) (-91.0002, -24.9649) (-90.9916, -25.935) (-91.3508, -26.9039) (-91.9897, -27.634) knots -1 -1 -1 -1 -0.506107 -0.506107 -0.506107 0 0 0 0
  spline S216 degree 3 poles (-91.9897, -17.634) (-92.7286, -18.4785) (-93.8364, -18.9881) (-94.9584, -18.9998) (-96.1081, -19.0117) (-97.2531, -18.4994) (-98.0103, -17.634) knots -1 -1 -1 -1 -0.506107 -0.506107 -0.506107 0 0 0 0
  spline S217 degree 3 poles (-98.0103, -17.634) (-98.6337, -16.9215) (-98.9915, -15.9818) (-98.9998, -15.0351) (-99.0084, -14.065) (-98.6492, -13.0961) (-98.0103, -12.366) knots -1 -1 -1 -1 -0.506107 -0.506107 -0.506107 0 0 0 0
  spline S218 degree 3 poles (-98.0103, -12.366) (-97.2714, -11.5215) (-96.1636, -11.0119) (-95.0416, -11.0002) (-93.8919, -10.9883) (-92.7469, -11.5006) (-91.9897, -12.366) knots -1 -1 -1 -1 -0.506107 -0.506107 -0.506107 0 0 0 0
  spline S219 degree 3 poles (-91.9897, -12.366) (-91.3663, -13.0785) (-91.0085, -14.0182) (-91.0002, -14.9649) (-90.9916, -15.935) (-91.3508, -16.9039) (-91.9897, -17.634) knots -1 -1 -1 -1 -0.506107 -0.506107 -0.506107 0 0 0 0
  spline S220 degree 3 poles (-91.9897, -7.634) (-92.7286, -8.4785) (-93.8364, -8.9881) (-94.9584, -8.9998) (-96.1081, -9.0117) (-97.2531, -8.4994) (-98.0103, -7.634) knots -1 -1 -1 -1 -0.506107 -0.506107 -0.506107 0 0 0 0
  spline S221 degree 3 poles (-98.0103, -7.634) (-98.6337, -6.9215) (-98.9915, -5.9818) (-98.9998, -5.0351) (-99.0084, -4.065) (-98.6492, -3.0961) (-98.0103, -2.366) knots -1 -1 -1 -1 -0.506107 -0.506107 -0.506107 0 0 0 0
  spline S222 degree 3 poles (-98.0103, -2.366) (-97.2714, -1.5215) (-96.1636, -1.0119) (-95.0416, -1.0002) (-93.8919, -0.9883) (-92.7469, -1.5006) (-91.9897, -2.366) knots -1 -1 -1 -1 -0.506107 -0.506107 -0.506107 0 0 0 0
  spline S223 degree 3 poles (-91.9897, -2.366) (-91.3663, -3.0785) (-91.0085, -4.0182) (-91.0002, -4.9649) (-90.9916, -5.935) (-91.3508, -6.9039) (-91.9897, -7.634) knots -1 -1 -1 -1 -0.506107 -0.506107 -0.506107 0 0 0 0
  spline S224 degree 3 poles (-81.9897, -77.634) (-82.7286, -78.4785) (-83.8364, -78.9881) (-84.9584, -78.9998) (-86.1081, -79.0117) (-87.2531, -78.4994) (-88.0103, -77.634) knots -1 -1 -1 -1 -0.506107 -0.506107 -0.506107 0 0 0 0
  spline S225 degree 3 poles (-88.0103, -77.634) (-88.6337, -76.9215) (-88.9915, -75.9818) (-88.9998, -75.0351) (-89.0084, -74.065) (-88.6492, -73.0961) (-88.0103, -72.366) knots -1 -1 -1 -1 -0.506107 -0.506107 -0.506107 0 0 0 0
  spline S226 degree 3 poles (-88.0103, -72.366) (-87.2714, -71.5215) (-86.1636, -71.0119) (-85.0416, -71.0002) (-83.8919, -70.9883) (-82.7469, -71.5006) (-81.9897, -72.366) knots -1 -1 -1 -1 -0.506107 -0.506107 -0.506107 0 0 0 0
  spline S227 degree 3 poles (-81.9897, -72.366) (-81.3663, -73.0785) (-81.0085, -74.0182) (-81.0002, -74.9649) (-80.9916, -75.935) (-81.3508, -76.9039) (-81.9897, -77.634) knots -1 -1 -1 -1 -0.506107 -0.506107 -0.506107 0 0 0 0
  spline S228 degree 3 poles (-81.9897, -67.634) (-82.7286, -68.4785) (-83.8364, -68.9881) (-84.9584, -68.9998) (-86.1081, -69.0117) (-87.2531, -68.4994) (-88.0103, -67.634) knots -1 -1 -1 -1 -0.506107 -0.506107 -0.506107 0 0 0 0
  spline S229 degree 3 poles (-88.0103, -67.634) (-88.6337, -66.9215) (-88.9915, -65.9818) (-88.9998, -65.0351) (-89.0084, -64.065) (-88.6492, -63.0961) (-88.0103, -62.366) knots -1 -1 -1 -1 -0.506107 -0.506107 -0.506107 0 0 0 0
  spline S230 degree 3 poles (-88.0103, -62.366) (-87.2714, -61.5215) (-86.1636, -61.0119) (-85.0416, -61.0002) (-83.8919, -60.9883) (-82.7469, -61.5006) (-81.9897, -62.366) knots -1 -1 -1 -1 -0.506107 -0.506107 -0.506107 0 0 0 0
  spline S231 degree 3 poles (-81.9897, -62.366) (-81.3663, -63.0785) (-81.0085, -64.0182) (-81.0002, -64.9649) (-80.9916, -65.935) (-81.3508, -66.9039) (-81.9897, -67.634) knots -1 -1 -1 -1 -0.506107 -0.506107 -0.506107 0 0 0 0
  spline S232 degree 3 poles (-81.9897, -57.634) (-82.7286, -58.4785) (-83.8364, -58.9881) (-84.9584, -58.9998) (-86.1081, -59.0117) (-87.2531, -58.4994) (-88.0103, -57.634) knots -1 -1 -1 -1 -0.506107 -0.506107 -0.506107 0 0 0 0
  spline S233 degree 3 poles (-88.0103, -57.634) (-88.6337, -56.9215) (-88.9915, -55.9818) (-88.9998, -55.0351) (-89.0084, -54.065) (-88.6492, -53.0961) (-88.0103, -52.366) knots -1 -1 -1 -1 -0.506107 -0.506107 -0.506107 0 0 0 0
  spline S234 degree 3 poles (-88.0103, -52.366) (-87.2714, -51.5215) (-86.1636, -51.0119) (-85.0416, -51.0002) (-83.8919, -50.9883) (-82.7469, -51.5006) (-81.9897, -52.366) knots -1 -1 -1 -1 -0.506107 -0.506107 -0.506107 0 0 0 0
  spline S235 degree 3 poles (-81.9897, -52.366) (-81.3663, -53.0785) (-81.0085, -54.0182) (-81.0002, -54.9649) (-80.9916, -55.935) (-81.3508, -56.9039) (-81.9897, -57.634) knots -1 -1 -1 -1 -0.506107 -0.506107 -0.506107 0 0 0 0
  spline S236 degree 3 poles (-81.9897, -47.634) (-82.7286, -48.4785) (-83.8364, -48.9881) (-84.9584, -48.9998) (-86.1081, -49.0117) (-87.2531, -48.4994) (-88.0103, -47.634) knots -1 -1 -1 -1 -0.506107 -0.506107 -0.506107 0 0 0 0
  spline S237 degree 3 poles (-88.0103, -47.634) (-88.6337, -46.9215) (-88.9915, -45.9818) (-88.9998, -45.0351) (-89.0084, -44.065) (-88.6492, -43.0961) (-88.0103, -42.366) knots -1 -1 -1 -1 -0.506107 -0.506107 -0.506107 0 0 0 0
  spline S238 degree 3 poles (-88.0103, -42.366) (-87.2714, -41.5215) (-86.1636, -41.0119) (-85.0416, -41.0002) (-83.8919, -40.9883) (-82.7469, -41.5006) (-81.9897, -42.366) knots -1 -1 -1 -1 -0.506107 -0.506107 -0.506107 0 0 0 0
  spline S239 degree 3 poles (-81.9897, -42.366) (-81.3663, -43.0785) (-81.0085, -44.0182) (-81.0002, -44.9649) (-80.9916, -45.935) (-81.3508, -46.9039) (-81.9897, -47.634) knots -1 -1 -1 -1 -0.506107 -0.506107 -0.506107 0 0 0 0
  spline S240 degree 3 poles (-81.9897, -37.634) (-82.7286, -38.4785) (-83.8364, -38.9881) (-84.9584, -38.9998) (-86.1081, -39.0117) (-87.2531, -38.4994) (-88.0103, -37.634) knots -1 -1 -1 -1 -0.506107 -0.506107 -0.506107 0 0 0 0
  spline S241 degree 3 poles (-88.0103, -37.634) (-88.6337, -36.9215) (-88.9915, -35.9818) (-88.9998, -35.0351) (-89.0084, -34.065) (-88.6492, -33.0961) (-88.0103, -32.366) knots -1 -1 -1 -1 -0.506107 -0.506107 -0.506107 0 0 0 0
  spline S242 degree 3 poles (-88.0103, -32.366) (-87.2714, -31.5215) (-86.1636, -31.0119) (-85.0416, -31.0002) (-83.8919, -30.9883) (-82.7469, -31.5006) (-81.9897, -32.366) knots -1 -1 -1 -1 -0.506107 -0.506107 -0.506107 0 0 0 0
  spline S243 degree 3 poles (-81.9897, -32.366) (-81.3663, -33.0785) (-81.0085, -34.0182) (-81.0002, -34.9649) (-80.9916, -35.935) (-81.3508, -36.9039) (-81.9897, -37.634) knots -1 -1 -1 -1 -0.506107 -0.506107 -0.506107 0 0 0 0
  spline S244 degree 3 poles (-81.9897, -27.634) (-82.7286, -28.4785) (-83.8364, -28.9881) (-84.9584, -28.9998) (-86.1081, -29.0117) (-87.2531, -28.4994) (-88.0103, -27.634) knots -1 -1 -1 -1 -0.506107 -0.506107 -0.506107 0 0 0 0
  spline S245 degree 3 poles (-88.0103, -27.634) (-88.6337, -26.9215) (-88.9915, -25.9818) (-88.9998, -25.0351) (-89.0084, -24.065) (-88.6492, -23.0961) (-88.0103, -22.366) knots -1 -1 -1 -1 -0.506107 -0.506107 -0.506107 0 0 0 0
  spline S246 degree 3 poles (-88.0103, -22.366) (-87.2714, -21.5215) (-86.1636, -21.0119) (-85.0416, -21.0002) (-83.8919, -20.9883) (-82.7469, -21.5006) (-81.9897, -22.366) knots -1 -1 -1 -1 -0.506107 -0.506107 -0.506107 0 0 0 0
  spline S247 degree 3 poles (-81.9897, -22.366) (-81.3663, -23.0785) (-81.0085, -24.0182) (-81.0002, -24.9649) (-80.9916, -25.935) (-81.3508, -26.9039) (-81.9897, -27.634) knots -1 -1 -1 -1 -0.506107 -0.506107 -0.506107 0 0 0 0
  spline S248 degree 3 poles (-81.9897, -17.634) (-82.7286, -18.4785) (-83.8364, -18.9881) (-84.9584, -18.9998) (-86.1081, -19.0117) (-87.2531, -18.4994) (-88.0103, -17.634) knots -1 -1 -1 -1 -0.506107 -0.506107 -0.506107 0 0 0 0
  spline S249 degree 3 poles (-88.0103, -17.634) (-88.6337, -16.9215) (-88.9915, -15.9818) (-88.9998, -15.0351) (-89.0084, -14.065) (-88.6492, -13.0961) (-88.0103, -12.366) knots -1 -1 -1 -1 -0.506107 -0.506107 -0.506107 0 0 0 0
  spline S250 degree 3 poles (-88.0103, -12.366) (-87.2714, -11.5215) (-86.1636, -11.0119) (-85.0416, -11.0002) (-83.8919, -10.9883) (-82.7469, -11.5006) (-81.9897, -12.366) knots -1 -1 -1 -1 -0.506107 -0.506107 -0.506107 0 0 0 0
  spline S251 degree 3 poles (-81.9897, -12.366) (-81.3663, -13.0785) (-81.0085, -14.0182) (-81.0002, -14.9649) (-80.9916, -15.935) (-81.3508, -16.9039) (-81.9897, -17.634) knots -1 -1 -1 -1 -0.506107 -0.506107 -0.506107 0 0 0 0
  spline S252 degree 3 poles (-81.9897, -7.634) (-82.7286, -8.4785) (-83.8364, -8.9881) (-84.9584, -8.9998) (-86.1081, -9.0117) (-87.2531, -8.4994) (-88.0103, -7.634) knots -1 -1 -1 -1 -0.506107 -0.506107 -0.506107 0 0 0 0
  spline S253 degree 3 poles (-88.0103, -7.634) (-88.6337, -6.9215) (-88.9915, -5.9818) (-88.9998, -5.0351) (-89.0084, -4.065) (-88.6492, -3.0961) (-88.0103, -2.366) knots -1 -1 -1 -1 -0.506107 -0.506107 -0.506107 0 0 0 0
  spline S254 degree 3 poles (-88.0103, -2.366) (-87.2714, -1.5215) (-86.1636, -1.0119) (-85.0416, -1.0002) (-83.8919, -0.9883) (-82.7469, -1.5006) (-81.9897, -2.366) knots -1 -1 -1 -1 -0.506107 -0.506107 -0.506107 0 0 0 0
  spline S255 degree 3 poles (-81.9897, -2.366) (-81.3663, -3.0785) (-81.0085, -4.0182) (-81.0002, -4.9649) (-80.9916, -5.935) (-81.3508, -6.9039) (-81.9897, -7.634) knots -1 -1 -1 -1 -0.506107 -0.506107 -0.506107 0 0 0 0
  spline S256 degree 3 poles (-71.9897, -77.634) (-72.7286, -78.4785) (-73.8364, -78.9881) (-74.9584, -78.9998) (-76.1081, -79.0117) (-77.2531, -78.4994) (-78.0103, -77.634) knots -1 -1 -1 -1 -0.506107 -0.506107 -0.506107 0 0 0 0
  spline S257 degree 3 poles (-78.0103, -77.634) (-78.6337, -76.9215) (-78.9915, -75.9818) (-78.9998, -75.0351) (-79.0084, -74.065) (-78.6492, -73.0961) (-78.0103, -72.366) knots -1 -1 -1 -1 -0.506107 -0.506107 -0.506107 0 0 0 0
  spline S258 degree 3 poles (-78.0103, -72.366) (-77.2714, -71.5215) (-76.1636, -71.0119) (-75.0416, -71.0002) (-73.8919, -70.9883) (-72.7469, -71.5006) (-71.9897, -72.366) knots -1 -1 -1 -1 -0.506107 -0.506107 -0.506107 0 0 0 0
  spline S259 degree 3 poles (-71.9897, -72.366) (-71.3663, -73.0785) (-71.0085, -74.0182) (-71.0002, -74.9649) (-70.9916, -75.935) (-71.3508, -76.9039) (-71.9897, -77.634) knots -1 -1 -1 -1 -0.506107 -0.506107 -0.506107 0 0 0 0
  spline S260 degree 3 poles (-71.9897, -67.634) (-72.7286, -68.4785) (-73.8364, -68.9881) (-74.9584, -68.9998) (-76.1081, -69.0117) (-77.2531, -68.4994) (-78.0103, -67.634) knots -1 -1 -1 -1 -0.506107 -0.506107 -0.506107 0 0 0 0
  spline S261 degree 3 poles (-78.0103, -67.634) (-78.6337, -66.9215) (-78.9915, -65.9818) (-78.9998, -65.0351) (-79.0084, -64.065) (-78.6492, -63.0961) (-78.0103, -62.366) knots -1 -1 -1 -1 -0.506107 -0.506107 -0.506107 0 0 0 0
  spline S262 degree 3 poles (-78.0103, -62.366) (-77.2714, -61.5215) (-76.1636, -61.0119) (-75.0416, -61.0002) (-73.8919, -60.9883) (-72.7469, -61.5006) (-71.9897, -62.366) knots -1 -1 -1 -1 -0.506107 -0.506107 -0.506107 0 0 0 0
  spline S263 degree 3 poles (-71.9897, -62.366) (-71.3663, -63.0785) (-71.0085, -64.0182) (-71.0002, -64.9649) (-70.9916, -65.935) (-71.3508, -66.9039) (-71.9897, -67.634) knots -1 -1 -1 -1 -0.506107 -0.506107 -0.506107 0 0 0 0
  spline S264 degree 3 poles (-71.9897, -57.634) (-72.7286, -58.4785) (-73.8364, -58.9881) (-74.9584, -58.9998) (-76.1081, -59.0117) (-77.2531, -58.4994) (-78.0103, -57.634) knots -1 -1 -1 -1 -0.506107 -0.506107 -0.506107 0 0 0 0
  spline S265 degree 3 poles (-78.0103, -57.634) (-78.6337, -56.9215) (-78.9915, -55.9818) (-78.9998, -55.0351) (-79.0084, -54.065) (-78.6492, -53.0961) (-78.0103, -52.366) knots -1 -1 -1 -1 -0.506107 -0.506107 -0.506107 0 0 0 0
  spline S266 degree 3 poles (-78.0103, -52.366) (-77.2714, -51.5215) (-76.1636, -51.0119) (-75.0416, -51.0002) (-73.8919, -50.9883) (-72.7469, -51.5006) (-71.9897, -52.366) knots -1 -1 -1 -1 -0.506107 -0.506107 -0.506107 0 0 0 0
  spline S267 degree 3 poles (-71.9897, -52.366) (-71.3663, -53.0785) (-71.0085, -54.0182) (-71.0002, -54.9649) (-70.9916, -55.935) (-71.3508, -56.9039) (-71.9897, -57.634) knots -1 -1 -1 -1 -0.506107 -0.506107 -0.506107 0 0 0 0
  spline S268 degree 3 poles (-71.9897, -47.634) (-72.7286, -48.4785) (-73.8364, -48.9881) (-74.9584, -48.9998) (-76.1081, -49.0117) (-77.2531, -48.4994) (-78.0103, -47.634) knots -1 -1 -1 -1 -0.506107 -0.506107 -0.506107 0 0 0 0
  spline S269 degree 3 poles (-78.0103, -47.634) (-78.6337, -46.9215) (-78.9915, -45.9818) (-78.9998, -45.0351) (-79.0084, -44.065) (-78.6492, -43.0961) (-78.0103, -42.366) knots -1 -1 -1 -1 -0.506107 -0.506107 -0.506107 0 0 0 0
  spline S270 degree 3 poles (-78.0103, -42.366) (-77.2714, -41.5215) (-76.1636, -41.0119) (-75.0416, -41.0002) (-73.8919, -40.9883) (-72.7469, -41.5006) (-71.9897, -42.366) knots -1 -1 -1 -1 -0.506107 -0.506107 -0.506107 0 0 0 0
  spline S271 degree 3 poles (-71.9897, -42.366) (-71.3663, -43.0785) (-71.0085, -44.0182) (-71.0002, -44.9649) (-70.9916, -45.935) (-71.3508, -46.9039) (-71.9897, -47.634) knots -1 -1 -1 -1 -0.506107 -0.506107 -0.506107 0 0 0 0
  spline S272 degree 3 poles (-71.9897, -37.634) (-72.7286, -38.4785) (-73.8364, -38.9881) (-74.9584, -38.9998) (-76.1081, -39.0117) (-77.2531, -38.4994) (-78.0103, -37.634) knots -1 -1 -1 -1 -0.506107 -0.506107 -0.506107 0 0 0 0
  spline S273 degree 3 poles (-78.0103, -37.634) (-78.6337, -36.9215) (-78.9915, -35.9818) (-78.9998, -35.0351) (-79.0084, -34.065) (-78.6492, -33.0961) (-78.0103, -32.366) knots -1 -1 -1 -1 -0.506107 -0.506107 -0.506107 0 0 0 0
  spline S274 degree 3 poles (-78.0103, -32.366) (-77.2714, -31.5215) (-76.1636, -31.0119) (-75.0416, -31.0002) (-73.8919, -30.9883) (-72.7469, -31.5006) (-71.9897, -32.366) knots -1 -1 -1 -1 -0.506107 -0.506107 -0.506107 0 0 0 0
  spline S275 degree 3 poles (-71.9897, -32.366) (-71.3663, -33.0785) (-71.0085, -34.0182) (-71.0002, -34.9649) (-70.9916, -35.935) (-71.3508, -36.9039) (-71.9897, -37.634) knots -1 -1 -1 -1 -0.506107 -0.506107 -0.506107 0 0 0 0
  spline S276 degree 3 poles (-71.9897, -27.634) (-72.7286, -28.4785) (-73.8364, -28.9881) (-74.9584, -28.9998) (-76.1081, -29.0117) (-77.2531, -28.4994) (-78.0103, -27.634) knots -1 -1 -1 -1 -0.506107 -0.506107 -0.506107 0 0 0 0
  spline S277 degree 3 poles (-78.0103, -27.634) (-78.6337, -26.9215) (-78.9915, -25.9818) (-78.9998, -25.0351) (-79.0084, -24.065) (-78.6492, -23.0961) (-78.0103, -22.366) knots -1 -1 -1 -1 -0.506107 -0.506107 -0.506107 0 0 0 0
  spline S278 degree 3 poles (-78.0103, -22.366) (-77.2714, -21.5215) (-76.1636, -21.0119) (-75.0416, -21.0002) (-73.8919, -20.9883) (-72.7469, -21.5006) (-71.9897, -22.366) knots -1 -1 -1 -1 -0.506107 -0.506107 -0.506107 0 0 0 0
  spline S279 degree 3 poles (-71.9897, -22.366) (-71.3663, -23.0785) (-71.0085, -24.0182) (-71.0002, -24.9649) (-70.9916, -25.935) (-71.3508, -26.9039) (-71.9897, -27.634) knots -1 -1 -1 -1 -0.506107 -0.506107 -0.506107 0 0 0 0
  spline S280 degree 3 poles (-71.9897, -17.634) (-72.7286, -18.4785) (-73.8364, -18.9881) (-74.9584, -18.9998) (-76.1081, -19.0117) (-77.2531, -18.4994) (-78.0103, -17.634) knots -1 -1 -1 -1 -0.506107 -0.506107 -0.506107 0 0 0 0
  spline S281 degree 3 poles (-78.0103, -17.634) (-78.6337, -16.9215) (-78.9915, -15.9818) (-78.9998, -15.0351) (-79.0084, -14.065) (-78.6492, -13.0961) (-78.0103, -12.366) knots -1 -1 -1 -1 -0.506107 -0.506107 -0.506107 0 0 0 0
  spline S282 degree 3 poles (-78.0103, -12.366) (-77.2714, -11.5215) (-76.1636, -11.0119) (-75.0416, -11.0002) (-73.8919, -10.9883) (-72.7469, -11.5006) (-71.9897, -12.366) knots -1 -1 -1 -1 -0.506107 -0.506107 -0.506107 0 0 0 0
  spline S283 degree 3 poles (-71.9897, -12.366) (-71.3663, -13.0785) (-71.0085, -14.0182) (-71.0002, -14.9649) (-70.9916, -15.935) (-71.3508, -16.9039) (-71.9897, -17.634) knots -1 -1 -1 -1 -0.506107 -0.506107 -0.506107 0 0 0 0
  spline S284 degree 3 poles (-71.9897, -7.634) (-72.7286, -8.4785) (-73.8364, -8.9881) (-74.9584, -8.9998) (-76.1081, -9.0117) (-77.2531, -8.4994) (-78.0103, -7.634) knots -1 -1 -1 -1 -0.506107 -0.506107 -0.506107 0 0 0 0
  spline S285 degree 3 poles (-78.0103, -7.634) (-78.6337, -6.9215) (-78.9915, -5.9818) (-78.9998, -5.0351) (-79.0084, -4.065) (-78.6492, -3.0961) (-78.0103, -2.366) knots -1 -1 -1 -1 -0.506107 -0.506107 -0.506107 0 0 0 0
  spline S286 degree 3 poles (-78.0103, -2.366) (-77.2714, -1.5215) (-76.1636, -1.0119) (-75.0416, -1.0002) (-73.8919, -0.9883) (-72.7469, -1.5006) (-71.9897, -2.366) knots -1 -1 -1 -1 -0.506107 -0.506107 -0.506107 0 0 0 0
  spline S287 degree 3 poles (-71.9897, -2.366) (-71.3663, -3.0785) (-71.0085, -4.0182) (-71.0002, -4.9649) (-70.9916, -5.935) (-71.3508, -6.9039) (-71.9897, -7.634) knots -1 -1 -1 -1 -0.506107 -0.506107 -0.506107 0 0 0 0
  spline S288 degree 3 poles (-61.9897, -77.634) (-62.7286, -78.4785) (-63.8364, -78.9881) (-64.9584, -78.9998) (-66.1081, -79.0117) (-67.2531, -78.4994) (-68.0103, -77.634) knots -1 -1 -1 -1 -0.506107 -0.506107 -0.506107 0 0 0 0
  spline S289 degree 3 poles (-68.0103, -77.634) (-68.6337, -76.9215) (-68.9915, -75.9818) (-68.9998, -75.0351) (-69.0084, -74.065) (-68.6492, -73.0961) (-68.0103, -72.366) knots -1 -1 -1 -1 -0.506107 -0.506107 -0.506107 0 0 0 0
  spline S290 degree 3 poles (-68.0103, -72.366) (-67.2714, -71.5215) (-66.1636, -71.0119) (-65.0416, -71.0002) (-63.8919, -70.9883) (-62.7469, -71.5006) (-61.9897, -72.366) knots -1 -1 -1 -1 -0.506107 -0.506107 -0.506107 0 0 0 0
  spline S291 degree 3 poles (-61.9897, -72.366) (-61.3663, -73.0785) (-61.0085, -74.0182) (-61.0002, -74.9649) (-60.9916, -75.935) (-61.3508, -76.9039) (-61.9897, -77.634) knots -1 -1 -1 -1 -0.506107 -0.506107 -0.506107 0 0 0 0
  spline S292 degree 3 poles (-61.9897, -67.634) (-62.7286, -68.4785) (-63.8364, -68.9881) (-64.9584, -68.9998) (-66.1081, -69.0117) (-67.2531, -68.4994) (-68.0103, -67.634) knots -1 -1 -1 -1 -0.506107 -0.506107 -0.506107 0 0 0 0
  spline S293 degree 3 poles (-68.0103, -67.634) (-68.6337, -66.9215) (-68.9915, -65.9818) (-68.9998, -65.0351) (-69.0084, -64.065) (-68.6492, -63.0961) (-68.0103, -62.366) knots -1 -1 -1 -1 -0.506107 -0.506107 -0.506107 0 0 0 0